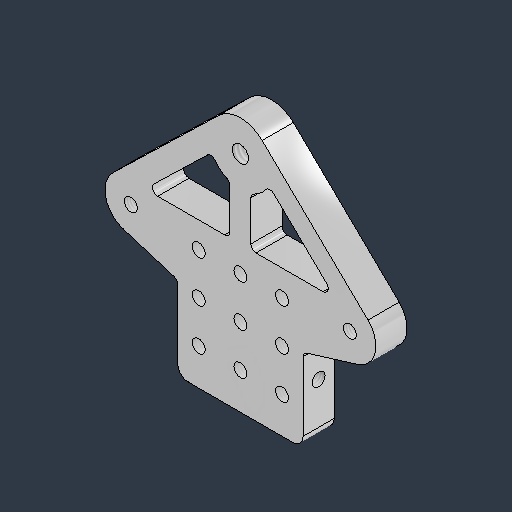
# Autodesk Inventor part: PLATE,TOP,ELEVATOR,STAGE1
Saved by Autodesk Inventor 2024.3 (Build 283343000, 343)
## iProperties
ILogicPurgeVersion: 0.0.0.0
OnSaveVersion: 3.4.3.0
OnSaveAssembly: COREAutomationManager
Created: 2025-01-27
Part Number: PLATE,TOP,ELEVATOR,STAGE1
Material: Aluminum 7075
Document SubType Name: Modeling
Designer: Jthib
Density: 2.81 g/cm^3
Appearance: Aluminum - Polished
Mfg Approved By: John.Thibert
Sheet Metal Rule: Default
Mass: 83.4067 g
Surface Area: 97.3008 cm^2
Volume: 29.6821 cm^3
ModelCat: Uncategorized
MaterialName: Aluminum 7075
CN_MASS: 0.08
Author: Jthib
Autodesk Inventor part; units mm, degrees
ref_plane "YZ Plane" through (0, 0, 0) normal (1, 0, 0) x (0, 1, 0)
ref_plane "XZ Plane" through (0, 0, 0) normal (0, 1, 0) x (-1, 0, 0)
ref_plane "XY Plane" through (0, 0, 0) normal (0, 0, 1) x (1, 0, 0)
sketch "Sketch1" plane through (0, 0, 0) normal (0, 0, 1) x (1, 0, 0)
  line L0 (33.401, 0) -> (-33.401, 0) construction
  arc A0 (38.9253, 5.6997) -> (35.7349, -7.5866) centre (33.401, 0) ccw construction
  arc A1 (-35.7349, -7.5866) -> (-38.9253, 5.6997) centre (-33.401, 0) ccw construction
  line L1 (19.1135, -12.7) -> (19.1135, -38.1)
  line L2 (-19.1135, -38.1) -> (-19.1135, -12.7)
  line L3 (-19.1135, -12.7) -> (-35.7349, -7.5866)
  arc A2 (35.7349, -7.5866) -> (38.9253, 5.6997) centre (33.401, 0) ccw
  arc A3 (-38.9253, 5.6997) -> (-35.7349, -7.5866) centre (-33.401, 0) ccw
  line L4 (0, 55.245) -> (0, -53.6575) construction
  line L5 (-19.1135, -38.1) -> (19.1135, -38.1)
  line L6 (35.7349, -7.5866) -> (19.1135, -12.7)
  line L7 (38.9253, 5.6997) -> (6.6291, 37.0021)
  circle A4 centre (0, 30.1625) radius 9.525
  line L8 (-6.6291, 37.0021) -> (-38.9253, 5.6997)
  line L9 (29.1304, 6.35) -> (8.6581, 26.1923)
  line L10 (3.175, 21.1822) -> (3.175, 6.35)
  line L11 (3.175, 6.35) -> (29.1304, 6.35)
  line L12 (-29.1304, 6.35) -> (-8.6581, 26.1923)
  line L13 (-3.175, 21.1822) -> (-3.175, 6.35)
  line L14 (-3.175, 6.35) -> (-29.1304, 6.35)
  point P0 (0, 0)
  point P1 (0, 0)
  point P2 (-8.6581, 26.1923)
  point P3 (-3.175, 21.1822)
  dimension "d24" = 50.927
  dimension "d25" = 7.9375
  dimension "d26" = 25.4
  dimension "d30" = 6.35
  dimension "d73" = 12.7
  dimension "d112" = 9.525
  dimension "d113" = 30.1625
  dimension "d115" = 6.35
  dimension "d116" = 6.35
  dimension "d117" = 6.35
  constraints: 29 end point, 13 point on circle, 6 tangent, 5 centre point, 5 coincident, 4 symmetric about line, 3 horizontal, 3 parallel, 2 vertical, 1 equal radius, 1 midpoint, 1 point on line, 1 other
  measures "d25" radius of A2
  measures "d26" distance of L1.start L1.end
  measures "d30" distance edge to line of A0 L1
  measures "d73" distance from line of L0 L1.start
  measures "d112" radius of A4
  measures "d113" distance from line of L0 A4.centre
  measures "d115" distance between parallel lines of L7 L9
  measures "d116" diameter of L10 L4
  measures "d117" distance between parallel lines of L0 L11
extrude "Extrusion2" add sketch "Sketch1" along normal mid plane 9.525 contours L1 L5 L2 L3 A3 L8 A4 L12 L14 L13 L10 L11 L9 L7 A2 L6 | A4
sketch "Sketch2" plane through (0, 0, 4.7625) normal (0, 0, 1) x (1, 0, 0)
  arc A0 (-38.9253, 5.6997) -> (-35.7349, -7.5866) centre (-33.401, 0) ccw construction
  line L0 (-33.401, 0) -> (33.401, 0) construction
  point P0 (0, 0)
  point P1 (0, 0)
  constraints: 3 coincident, 2 end point, 1 horizontal, 1 midpoint
hole "Hole1" at (33.401, 0, 4.7625) at (-33.401, 0, 4.7625) direction (0, 0, -1) diameter 3.9624 end through all start extended yes thread size "10-32 UNF" class "2B" standard "ANSI Unified Screw Threads"
sketch "Sketch3" plane through (0, 0, -4.7625) normal (0, 0, -1) x (-1, 0, 0)
  line L0 (-57.8739, 0) -> (57.8739, 0) construction
  line L1 (0, -53.6575) -> (0, 55.245) construction
  line L2 (12.7, -1.5875) -> (-12.7, -1.5875) construction
  line L3 (12.7, -14.2875) -> (-12.7, -14.2875) construction
  line L4 (12.7, -26.9875) -> (-12.7, -26.9875) construction
  point P0 (0, 0)
  point P1 (0, -1.5875)
  point P2 (0, -14.2875)
  point P3 (0, -26.9875)
  dimension "d43" = 25.4
  dimension "d45" = 1.5875
  dimension "d107" = 12.7
  constraints: 6 end point, 2 coincident, 1 horizontal, 1 midpoint, 1 point on line, 1 vertical, 8 other
  measures "d43" distance of L2.start L2.end
  measures "d45" distance between parallel lines of L0 L2
  measures "d107" distance of L2.start L3.start
hole "Hole2" at (12.7, -1.5875, -4.7625) at (-12.7, -1.5875, -4.7625) at (0, -1.5875, -4.7625) at (12.7, -14.2875, -4.7625) at (0, -14.2875, -4.7625) at (-12.7, -14.2875, -4.7625) at (12.7, -26.9875, -4.7625) at (0, -26.9875, -4.7625) at (-12.7, -26.9875, -4.7625) direction (0, 0, 1) diameter 3.9624 end through all thread size "10-32 UNF" class "2B" standard "ANSI Unified Screw Threads"
sketch "Sketch6" plane through (19.1135, -38.1, 4.7625) normal (1, 0, 0) x (0, 0, -1)
  line L0 (9.525, 25.4) -> (0, 25.4) construction
  line L1 (0, 0) -> (0, 25.4) construction
  line L2 (9.525, 25.4) -> (9.525, 0) construction
  line L3 (9.525, 0) -> (0, 0) projected
  point P0 (4.7625, 38.1)
  point P1 (4.7625, 15.875)
  dimension "d74" = 22.225
  constraints: 1 vertical alignment
  measures "d74" distance of point (4.763, 15.875) point (4.763, 38.1)
hole "Hole3" at (19.1135, -22.225, 0) direction (-1, 0, 0) diameter 3.9624 end through all thread size "10-32 UNF" class "2B" standard "ANSI Unified Screw Threads"
sketch "Sketch7" plane through (0, 0, 4.7625) normal (0, 0, 1) x (1, 0, 0)
  arc A0 (6.6291, 37.0021) -> (-6.6291, 37.0021) centre (0, 30.1625) ccw construction
  point P0 (0, 0)
  constraints: 1 coincident
hole "Hole4" at (0, 30.1625, 4.7625) direction (0, 0, -1) diameter 4.9784 end through all thread size "1/4-20 UNC" class "2B" standard "ANSI Unified Screw Threads"
fillet "Fillet5" radius 3.175 2 edges at (-19.1135, -38.1, 0) (19.1135, -38.1, 0)
fillet "Fillet7" radius 1.5875 10 edges at (-19.1135, -12.7, 0) (19.1135, -12.7, 0) (29.1304, 6.35, 0) (3.175, 6.35, 0) (3.175, 21.1822, 0) (8.6581, 26.1923, 0) (-3.175, 21.1822, 0) (-8.6581, 26.1923, 0) (-3.175, 6.35, 0) (-29.1304, 6.35, 0)
equation "\"BendRadius\" = Thickness"
equation "\"BendReliefWidth\" = Thickness"
equation "\"BendReliefDepth\" = 0.5 * Thickness"
equation "\"CornerReliefSize\" = 4 * Thickness"
equation "\"MinimumRemnant\" = 2 * Thickness"
equation "\"TransitionRadius\" = BendRadius"
equation "\"JacobiRadiusSize\" = BendRadius"
equation "\"GapSize\" = Thickness"
equation "\"Thickness\" = 6.35"
body "Solid3"
